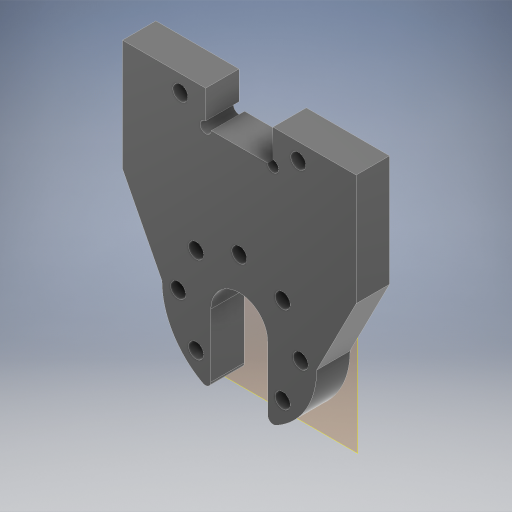
# Autodesk Inventor part: leg_between
Saved by Autodesk Inventor 2024 (Build 280153000, 153)
## iProperties
Created: 2024-09-03
Part Number: leg_between
Material: PMMA 플라스틱
Document SubType Name: Modeling
Designer: msi
Density: 1.188 g/cm^3
Appearance: 매끄러움 - 검은색
Author: msi
Autodesk Inventor part; units mm, degrees
ref_plane "YZ Plane" through (0, 0, 0) normal (1, 0, 0) x (0, 1, 0)
ref_plane "XZ Plane" through (0, 0, 0) normal (0, 1, 0) x (-1, 0, 0)
ref_plane "XY Plane" through (0, 0, 0) normal (0, 0, 1) x (1, 0, 0)
ref_plane "작업 평면1" through (0, 0, 0) normal (0, 0, 1) x (1, 0, 0)
sketch "스케치1" plane through (0, 0, 0) normal (0, 0, 1) x (1, 0, 0)
  circle A0 centre (-7.7782, -7.7782) radius 1.55 projected
  circle A1 centre (7.7782, -7.7782) radius 1.55 projected
  circle A2 centre (7.7782, 7.7782) radius 1.55 projected
  circle A3 centre (-7.7782, 7.7782) radius 1.55 projected
  circle A4 centre (0, 0) radius 5 projected
  circle A5 centre (0, 0) radius 13.9 projected
  circle A6 centre (0, 11) radius 1.55 projected
  circle A7 centre (11, 0) radius 1.55 projected
  circle A8 centre (0, -11) radius 1.55 projected
  circle A9 centre (-11, 0) radius 1.55 projected
  circle A10 centre (11, 0) radius 1.35
  circle A11 centre (7.7782, 7.7782) radius 1.35
  circle A12 centre (0, 11) radius 1.35
  circle A13 centre (-7.7782, 7.7782) radius 1.35
  circle A14 centre (-11, 0) radius 1.35
  circle A15 centre (-7.7782, -7.7782) radius 1.35
  circle A16 centre (0, -11) radius 1.35
  circle A17 centre (7.7782, -7.7782) radius 1.35
  line L0 (13.9, 33.9052) -> (-13.9, 33.9052)
  line L1 (-3.1, 33.9052) -> (3.1, 33.9052)
  circle A18 centre (0, 0) radius 5.1
  circle A19 centre (0, 0) radius 13.9
  line L2 (-5.1, 0) -> (-5.1, -12.9306)
  line L3 (5.1, 0) -> (5.1, -12.9306)
  line L4 (13.9, 33.9052) -> (21, 33.9052)
  line L5 (21, 33.9052) -> (21, 13.9)
  line L6 (13.9, 13.9) -> (13.9, 13.9052)
  line L7 (-13.9, 33.9052) -> (-21, 33.9052)
  line L8 (-21, 33.9052) -> (-21, 13.9)
  line L9 (21, 13.9) -> (13.9, 0)
  line L10 (-21, 13.9) -> (-13.9, 0)
  line L11 (6.05, 33.9052) -> (-6.05, 33.9052)
  line L12 (-6.05, 33.9052) -> (-6.05, 27.8052)
  line L13 (-6.05, 27.8052) -> (6.05, 27.8052)
  line L14 (6.05, 27.8052) -> (6.05, 33.9052)
  circle A20 centre (10.6, 30.905) radius 1.35
  circle A21 centre (-10.6, 30.905) radius 1.35
  point P0 (13.9, 0)
  dimension "d1" = 2.7
  dimension "d4" = 360
  dimension "d34" = 0.1
  dimension "d37" = 12.1
  dimension "d38" = 6.1
  dimension "d44" = 2.7
  dimension "d45" = 2.7
  constraints: 30 end point, 12 centre point, 4 horizontal, 4 parallel, 4 point on circle, 3 perpendicular, 2 coincident, 2 point on line, 2 tangent, 1 vertical, 20 other
  measures "d1" diameter of A10
  measures "d34" radial gap between concentric circles of A4 A18
  measures "d37" distance of L13.end L12.end
  measures "d38" distance of L12.end L11.end
  measures "d44" diameter of A20
  measures "d45" diameter of A21
extrude "돌출8" add sketch "스케치1" along normal blind 6 contours A0 | A1 | A2 | A3 | A5 L3 A18 L2 | A5 L10 L8 L7 L0 L12 L13 L14 L4 L5 L9 | A6 | A7 | A9 picked at (-7.5104, -2.4224)
fillet "모깎기2" radius 1 2 edges at (5.1, -12.9306, 3) (-5.1, -12.9306, 3)
sketch "스케치3" plane through (0, 0, 6) normal (0, 0, 1) x (1, 0, 0)
  line L0 (-6.05, 27.8052) -> (-6.05, 33.9052) projected
  line L1 (6.05, 27.8052) -> (-6.05, 27.8052) projected
  line L2 (6.05, 33.9052) -> (6.05, 27.8052) projected
  circle A0 centre (-6.05, 27.8052) radius 1
  circle A1 centre (6.05, 27.8052) radius 1
  point P0 (0, 0)
  dimension "d49" = 2
  dimension "d50" = 2
  constraints: 2 centre point, 2 coincident
  measures "d49" diameter of A0
  measures "d50" diameter of A1
extrude "돌출9" cut sketch "스케치3" against normal blind 10
